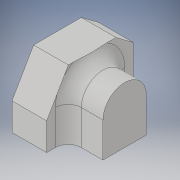
# Autodesk Inventor part: 410571040示範二
Saved by Autodesk Inventor 2017 (Build 210142000, 142)
## iProperties
Part Number: 410571040示範二
Material: 一般
Document SubType Name: Modeling
Designer: user
Density: 1 g/cm^3
Appearance: 預設
Author: user
Autodesk Inventor part; units mm, degrees
ref_plane "YZ Plane" through (0, 0, 0) normal (1, 0, 0) x (0, 1, 0)
ref_plane "XZ Plane" through (0, 0, 0) normal (0, 1, 0) x (-1, 0, 0)
ref_plane "XY Plane" through (0, 0, 0) normal (0, 0, 1) x (1, 0, 0)
sketch "草圖1" plane through (0, 0, 0) normal (1, 0, 0) x (0, 1, 0)
  line L0 (0, 0) -> (6.3397, 0)
  line L1 (6.3397, 0) -> (15, -5)
  line L2 (15, -5) -> (15, -16)
  line L3 (15, -16) -> (12, -20)
  line L4 (12, -20) -> (0, -20)
  line L5 (0, -20) -> (0, 0)
  dimension "d0" = 15
  dimension "d1" = 20
  dimension "d2" = 60
  dimension "d3" = 5
  dimension "d4" = 4
  dimension "d5" = 3
  constraints: 12 end point, 2 perpendicular, 1 horizontal, 1 parallel
  measures "d0" distance from line of L5 L1.end
  measures "d1" distance of L4.end L0.start
  measures "d2" angle of L2 L1
  measures "d3" distance from line of L1.end L0
  measures "d4" vertical distance of L3.end L2.end
  measures "d5" distance from line of L3.end L2
extrude "擠出1" add sketch "草圖1" along normal blind 8
sketch "草圖2" plane through (8, 0, 0) normal (1, 0, 0) x (0, 0, -1)
  line L0 (0, 0) -> (20, 0) projected
  line L1 (15, 0) -> (15, 8)
  arc A0 (15, 8) -> (5, 8) centre (10, 8) ccw
  line L2 (5, 8) -> (5, 0)
  line L3 (5, 8) -> (16.8472, 8) construction
  line L4 (10, 8) -> (10, 12.4145) construction
  line L5 (0, 6.3397) -> (0, 0) projected
  line L6 (5, 0) -> (15, 0)
  dimension "d8" = 10
  dimension "d9" = 5
  dimension "d10" = 8
  constraints: 10 end point, 3 point on line, 2 point on circle, 2 vertical, 1 centre point, 1 collinear, 1 horizontal, 1 perpendicular, 1 tangent
  measures "d8" distance between parallel lines of L4 L5
  measures "d9" radius of A0
  measures "d10" distance of L1.start L1.end
extrude "擠出2" add sketch "草圖2" along normal blind 8
fillet "圓角1" radius 3 3 edges at (8, 13, -10) (8, 4, -15) (8, 4, -5)
